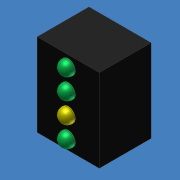
# Autodesk Inventor part: cRIO-FRC LED
Saved by Autodesk Inventor 2011 (Build 150239000, 239)
## iProperties
Category: FRC Parts
Manager: Ed Sparks
Company: FirstCadLibrary
Shininess: 64.0
Length Units: 11272
Angle Units: 11279
Time Units: 11290
Mass Units: 11286
Length Display Precision: 3
Angle Display Precision: 2
Compacted: True
Part Number: cRIO-FRC LED
Document SubType Name: Modeling
Created: 2008-12-13
Designer: Ed Sparks
Project: FIRST
Catalog Web Link: www.firstcadlibrary.com
Engineer: Ed Sparks
Density: 1 g/cm^3
Density: 0.0
Volumn: 0.0
Area: 0.0
PropertySet Name: Model Information
Control State: 0
Master: False
Checked Out: False
Author: Ed Sparks
Keywords: FIRST
Autodesk Inventor part; units mm, degrees
ref_plane "YZ Plane" through (0, 0, 0) normal (1, 0, 0) x (0, 1, 0)
ref_plane "XZ Plane" through (0, 0, 0) normal (0, 1, 0) x (-1, 0, 0)
ref_plane "XY Plane" through (0, 0, 0) normal (0, 0, 1) x (1, 0, 0)
sketch "Sketch1" plane through (0, 0, 0) normal (0, 0, 1) x (1, 0, 0)
  line L0 (-3.81, 5.08) -> (3.81, 5.08)
  line L1 (3.81, 5.08) -> (3.81, -5.08)
  line L2 (3.81, -5.08) -> (-3.81, -5.08)
  line L3 (-3.81, -5.08) -> (-3.81, 5.08)
  line L4 (0, 0) -> (0, 5.08) construction
  line L5 (0, 0) -> (0, -5.08) construction
  line L6 (0, 0) -> (-3.81, 0) construction
  line L7 (0, 0) -> (3.81, 0) construction
  dimension "d0" = 7.62
  dimension "d1" = 10.16
  constraints: 16 end point, 4 midpoint, 2 collinear, 2 parallel, 1 horizontal, 1 perpendicular, 1 other
  measures "d0" distance of L0.start L0.end
  measures "d1" distance of L2.end L0.start
extrude "Extrusion1" add sketch "Sketch1" along normal mid plane 6.35
sketch "Sketch2" plane through (0, 0, 3.175) normal (0, 0, 1) x (1, 0, 0)
  line L0 (-3.81, 5.08) -> (3.81, 5.08) projected
  line L1 (3.81, -5.08) -> (-3.81, -5.08) projected
  line L2 (0, 5.08) -> (0, -5.08) construction
  circle A0 centre (0, 3.81) radius 0.889
  line L3 (-3.81, -5.08) -> (-3.81, 5.08) projected
  circle A1 centre (0, 1.27) radius 0.889
  circle A2 centre (0, -1.27) radius 0.889
  circle A3 centre (0, -3.81) radius 0.889
  dimension "d4" = 1.27
  dimension "d5" = 1.778
  dimension "d14" = 2.54
  constraints: 4 centre point, 2 end point, 2 midpoint, 1 point on line, 1 vertical, 6 other
  measures "d4" distance from line of L0 A0.centre
  measures "d5" diameter of A0
  measures "d14" distance of A0.centre A1.centre
extrude "Extrusion2" add sketch "Sketch2" along normal blind 1.016 contours A0
fillet "Fillet1" radius 0.889 1 edges at (-0.889, 3.81, 4.191)
extrude "Extrusion3" add sketch "Sketch2" along normal blind 1.016 contours A1
fillet "Fillet2" radius 0.889 1 edges at (-0.889, 1.27, 4.191)
extrude "Extrusion4" add sketch "Sketch2" along normal blind 1.016 contours A2
fillet "Fillet3" radius 0.889 1 edges at (-0.889, -1.27, 4.191)
extrude "Extrusion5" add sketch "Sketch2" along normal blind 1.016 contours A3
fillet "Fillet4" radius 0.889 1 edges at (-0.889, -3.81, 4.191)
body "Solid1"
